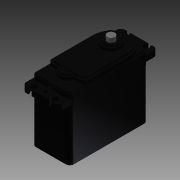
# Autodesk Inventor part: Quarter_scale_servo
Saved by Autodesk Inventor 2015 (Build 190159000, 159)
## iProperties
Created: 2013-11-11
Part Number: Quarter_scale_servo
Material: ABS Plastic
Document SubType Name: Modeling
Designer: 14hensgenw
Density: 1.06 g/cm^3
Appearance: Fine Textured - Black
Author: 14hensgenw
Autodesk Inventor part; units mm, degrees
ref_plane "YZ Plane" through (0, 0, 0) normal (1, 0, 0) x (0, 1, 0)
ref_plane "XZ Plane" through (0, 0, 0) normal (0, 1, 0) x (-1, 0, 0)
sketch "Sketch1" plane through (0, 0, 0) normal (1, 0, 0) x (0, 1, 0)
  line L0 (18.5394, 20.6785) -> (-27.9934, 20.6785)
  line L1 (-27.9934, 20.6785) -> (-27.9934, -37.9701)
  line L2 (-27.9934, -37.9701) -> (18.5394, -37.9701)
  line L3 (18.5394, -37.9701) -> (18.5394, 20.6785)
  point P0 (0, 0)
  dimension "d0" = 58.6486
  dimension "d1" = 46.5328
  constraints: 8 end point, 2 parallel, 1 horizontal, 1 perpendicular
  measures "d0" distance of L2.end L0.start
  measures "d1" distance of L0.start L0.end
extrude "Extrusion1" add sketch "Sketch1" along normal blind 28.4734
sketch "Sketch2" plane through (0, 18.5394, 20.6785) normal (0, 1, 0) x (1, 0, 0)
  line L0 (0, 58.6486) -> (0, 0) projected
  line L1 (0, 0) -> (28.4734, 0) projected
  line L2 (28.4734, 58.6486) -> (28.4734, 0) projected
  line L3 (0, 58.6486) -> (28.4734, 58.6486) projected
  line L4 (1.0287, 58.0708) -> (27.4447, 58.0708)
  line L5 (27.4447, 58.0708) -> (27.4447, 0.5778)
  line L6 (27.4447, 0.5778) -> (1.0287, 0.5778)
  line L7 (1.0287, 0.5778) -> (1.0287, 58.0708)
  line L8 (1.0287, 58.0708) -> (0, 58.0708)
  line L9 (27.4447, 58.0708) -> (28.4734, 58.0708)
  line L10 (14.2367, 58.6486) -> (14.2367, 58.0708)
  line L11 (15.3559, 0) -> (15.3559, 0.5778)
  point P0 (0, 20.6785)
  dimension "d4" = 26.416
  dimension "d5" = 57.4929
  constraints: 16 end point, 4 perpendicular, 4 point on line, 2 equal length, 2 midpoint, 2 parallel, 1 horizontal
  measures "d4" distance of L4.start L4.end
  measures "d5" distance between parallel lines of L6 L4
extrude "Extrusion2" cut sketch "Sketch2" against normal blind 1.016 contours L3 L10 L4 L8 L0 | L8 L7 L6 L11 L1 L0 | L3 L2 L9 L4 L10 | L11 L6 L5 L9 L2 L1
sketch "Sketch3" plane through (1.0287, 18.5394, 20.1007) normal (0, 1, 0) x (1, 0, 0)
  line L0 (0, 0) -> (26.416, 0) projected
  line L1 (0, 57.4929) -> (0, 0) projected
  line L2 (26.416, 57.4929) -> (0, 57.4929) projected
  line L3 (26.416, 0) -> (26.416, 57.4929) projected
  line L4 (27.4447, -0.5778) -> (-1.0287, -0.5778) projected
  line L5 (27.4447, 58.0708) -> (27.4447, -0.5778) projected
  line L6 (-1.0287, 58.0708) -> (27.4447, 58.0708) projected
  line L7 (-1.0287, -0.5778) -> (-1.0287, 58.0708) projected
  circle A0 centre (13.208, 44.4941) radius 13.5767
  line L8 (-0.3683, 44.5981) -> (-1.0287, 44.5981)
  line L9 (26.7843, 44.5981) -> (27.4447, 44.5981)
  line L10 (0, -0.5778) -> (0, 10.8268)
  line L11 (0, 10.8268) -> (-1.0287, 10.8268)
  line L12 (27.4447, 10.8268) -> (-1.0287, 10.8268)
  line L13 (-0.3683, 44.5981) -> (-0.3683, 10.8268)
  line L14 (26.7843, 44.5981) -> (26.7843, 10.8268)
  circle A1 centre (13.208, 12.2237) radius 6.1976
  line L15 (13.208, 10.8268) -> (13.208, 6.0262)
  line L16 (13.208, 6.0262) -> (13.208, 12.2237)
  point P0 (-1.0287, 20.1007)
  dimension "d12" = 12.3952
  dimension "d9" = 0.6604
  dimension "d10" = 11.4046
  dimension "d13" = 4.8006
  constraints: 18 end point, 8 point on line, 6 perpendicular, 2 collinear, 2 point on circle, 1 centre point, 1 midpoint, 1 parallel, 1 tangent, 1 vertical alignment, 2 other
  measures "d9" distance of L8.start L8.end
  measures "d10" distance of L10.start L10.end
  measures "d13" distance of L15.start L15.end
extrude "Extrusion3" add sketch "Sketch3" along normal blind 2.1209 contours L11 L13 A0 L1 | L1 A0 L3 L12 A1 | L3 A0 L14 L12 | A0 L1 | L1 A0 L2 L3 | A1 L12 | L12 L15 A1 | L3 A0 | A1 L15 L12 | A0 L2
sketch "Sketch4" plane through (1.0287, 20.6603, 20.1007) normal (0, 1, 0) x (1, 0, 0)
  line L0 (19.2461, 10.8268) -> (26.7843, 10.8268) projected
  line L1 (26.7843, 10.8268) -> (26.7843, 44.5981) projected
  arc A0 (26.7843, 44.5981) -> (-0.3683, 44.5981) centre (13.208, 44.4941) ccw projected
  line L2 (-0.3683, 44.5981) -> (-0.3683, 10.8268) projected
  line L3 (-0.3683, 10.8268) -> (7.1699, 10.8268) projected
  arc A1 (7.1699, 10.8268) -> (19.2461, 10.8268) centre (13.208, 12.2237) ccw projected
  arc A2 (25.4571, 44.5929) -> (0.9588, 44.5929) centre (13.208, 44.4941) ccw
  line L4 (25.4571, 44.5929) -> (25.4571, 12.1539)
  line L5 (25.4571, 12.1539) -> (18.0779, 12.1539)
  arc A3 (8.3381, 12.1539) -> (18.0779, 12.1539) centre (13.208, 12.2237) ccw
  line L6 (8.3381, 12.1539) -> (0.9588, 12.1539)
  line L7 (0.9588, 12.1539) -> (0.9588, 44.5929)
  point P0 (-1.0287, 20.1007)
  dimension "d18" = 24.4983
  constraints: 8 end point, 4 point on circle, 2 centre point, 5 other
  measures "d18" distance between parallel lines of L4 L7
extrude "Extrusion4" add sketch "Sketch4" along normal blind 1.1176 contours L4 L5 A3 L6 L7 A2
sketch "Sketch5" plane through (1.0287, 21.7779, 20.1007) normal (0, 1, 0) x (1, 0, 0)
  arc A0 (8.3381, 12.1539) -> (18.0779, 12.1539) centre (13.208, 12.2237) ccw projected
  line L0 (25.4571, 12.1539) -> (25.4571, 44.5929) projected
  line L1 (8.3381, 12.1539) -> (18.0779, 12.1539)
  arc A1 (8.3381, 12.1539) -> (18.0779, 12.1539) centre (13.208, 12.2237) ccw
  point P0 (-1.0287, 20.1007)
  constraints: 2 end point, 2 point on circle, 1 centre point, 1 concentric, 1 perpendicular
extrude "Extrusion5" cut sketch "Sketch5" against normal blind 0.4445
fillet "Fillet1" radius 3.175 12 edges at (27.4447, 18.0314, 20.1007) (27.813, 19.5998, 9.2739) (26.4859, 21.2191, 7.9468) (1.9876, 21.2191, 7.9468) (0.6604, 19.5998, 9.2739) (1.0287, 18.0314, 20.1007) (1.0287, 18.0314, -37.3922) (27.4447, 18.0314, -37.3922) (28.4734, -5.235, -37.9701) (28.4734, -5.235, 20.6785) (0, -5.235, -37.9701) (0, -5.235, 20.6785)
ref_plane "Work Plane1" through (0, 14.9072, 20.6785) normal (0, 1, 0) x (1, 0, 0)
sketch "Sketch6" plane through (0, 14.9072, 20.6785) normal (0, 1, 0) x (1, 0, 0)
  arc A0 (0, 3.175) -> (3.175, 0) centre (3.175, 3.175) ccw projected
  line L0 (0, 3.175) -> (0, 55.4736) projected
  arc A1 (3.175, 58.6486) -> (0, 55.4736) centre (3.175, 55.4736) ccw projected
  line L1 (3.175, 58.6486) -> (25.2984, 58.6486) projected
  arc A2 (28.4734, 55.4736) -> (25.2984, 58.6486) centre (25.2984, 55.4736) ccw projected
  line L2 (28.4734, 3.175) -> (28.4734, 55.4736) projected
  arc A3 (25.2984, 0) -> (28.4734, 3.175) centre (25.2984, 3.175) ccw projected
  line L3 (3.175, 0) -> (25.2984, 0) projected
  line L4 (0.3746, 66.2432) -> (28.0988, 66.2432)
  line L5 (28.0988, 66.2432) -> (28.0988, -7.5946)
  line L6 (28.0988, -7.5946) -> (0.3747, -7.5946)
  line L7 (0.3747, -7.5946) -> (0.3746, 66.2432)
  line L8 (14.2367, 58.6486) -> (14.2367, 0)
  line L9 (0.3747, 29.3243) -> (28.0987, 29.3243)
  line L10 (14.2367, -7.5946) -> (14.2367, 29.3243)
  point P0 (0, 20.6785)
  point P1 (14.2367, 29.3243)
  dimension "d23" = 27.7241
  dimension "d24" = 73.8378
  constraints: 14 end point, 7 midpoint, 2 parallel, 1 horizontal, 1 perpendicular
  measures "d23" distance between parallel lines of L5 L7
  measures "d24" distance of L4.end L5.end
extrude "Extrusion6" add sketch "Sketch6" against normal blind 4.0005 contours L7 L9 L8 L3 A0 | A0 L3 L10 L6 L7 | L7 A1 L1 L8 L9 | L7 L4 L5 A2 L1 A1 | L8 L9 L5 A3 L3 | L3 A3 L5 L6 L10 | L8 L1 A2 L5 L9
fillet "Fillet2" radius 3.175 4 edges at (28.0988, 12.9069, 28.2731) (0.3747, 12.9069, 28.2731) (0.3746, 12.9069, -45.5647) (28.0988, 12.9069, -45.5647)
sketch "Sketch7" plane through (0, 14.9072, 20.6785) normal (0, 1, 0) x (1, 0, 0)
  line L0 (3.5497, -7.5946) -> (24.9238, -7.5946) projected
  line L1 (28.0988, -4.4196) -> (28.0988, 1.6788) projected
  line L2 (3.175, 0) -> (25.2984, 0) projected
  line L3 (0.3746, 1.6788) -> (0.3747, -4.4196) projected
  line L4 (4.1592, 0) -> (4.1593, -7.5946)
  line L5 (24.3142, -7.5946) -> (24.3142, 0)
  line L6 (0.3747, -2.5273) -> (28.0988, -2.5273)
  circle A0 centre (6.3183, -4.6863) radius 2.159
  circle A1 centre (22.1552, -4.6863) radius 2.159
  point P0 (0, 20.6785)
  dimension "d28" = 3.7846
  dimension "d29" = 3.7846
  dimension "d30" = 5.0673
  dimension "d31" = 4.318
  dimension "d32" = 4.318
  constraints: 6 end point, 6 point on line, 4 tangent, 3 perpendicular, 2 centre point
  measures "d28" distance between parallel lines of L3 L4
  measures "d29" distance between parallel lines of L1 L5
  measures "d30" distance between parallel lines of L0 L6
  measures "d31" diameter of A0
  measures "d32" diameter of A1
extrude "Extrusion7" cut sketch "Sketch7" against normal blind 4.0005 contours A0 | A1
sketch "Sketch8" plane through (0, 14.9072, 20.6785) normal (0, 1, 0) x (1, 0, 0)
  circle A0 centre (6.3183, -4.6863) radius 2.159 projected
  arc A1 (0.3747, -4.4196) -> (3.5497, -7.5946) centre (3.5497, -4.4196) ccw projected
  line L0 (3.5497, -7.5946) -> (24.9238, -7.5946) projected
  line L1 (3.175, 0) -> (25.2984, 0) projected
  line L2 (0.3746, 1.6788) -> (0.3747, -4.4196) projected
  line L3 (0.3747, -4.4196) -> (0.3747, -8.9936)
  line L4 (0.3747, -7.5946) -> (5.0483, -7.5946)
  line L5 (5.0483, -7.5946) -> (5.0483, -6.4323)
  line L6 (5.0483, -7.5946) -> (7.6772, -7.5946)
  line L7 (7.6772, -7.5946) -> (7.6772, -6.364)
  arc A2 (5.0483, -6.4323) -> (7.6772, -6.364) centre (6.3183, -4.6863) ccw
  line L8 (14.2367, -7.5946) -> (14.2367, 0)
  circle A3 centre (22.1552, -4.6863) radius 2.159
  line L9 (24.9238, -7.5946) -> (3.5497, -7.5946)
  line L10 (28.0988, -7.5946) -> (23.4252, -7.5946)
  line L11 (23.4252, -7.5946) -> (23.4251, -6.4323)
  line L12 (23.4252, -7.5946) -> (20.7963, -7.5946)
  line L13 (20.7963, -7.5946) -> (20.7962, -6.364)
  arc A4 (20.7962, -6.364) -> (23.4251, -6.4323) centre (22.1552, -4.6863) ccw
  point P0 (0, 20.6785)
  dimension "d35" = 4.6736
  dimension "d36" = 2.6289
  constraints: 22 end point, 9 symmetric about line, 8 point on circle, 5 point on line, 3 centre point, 2 midpoint, 2 perpendicular, 1 collinear, 1 concentric, 1 tangent, 2 other
  measures "d35" distance of L4.start L4.end
  measures "d36" distance of L4.end L6.end
extrude "Extrusion8" cut sketch "Sketch8" against normal blind 4.0005 contours A0 L7 L0 L5 | L13 A3 L11 L0
sketch "Sketch9" plane through (0, 14.9072, 20.6785) normal (0, 1, 0) x (1, 0, 0)
  line L0 (7.6772, -7.5946) -> (20.7963, -7.5946) projected
  line L1 (3.175, 0) -> (25.2984, 0) projected
  line L2 (14.2367, 0) -> (14.2367, -7.5946)
  circle A0 centre (14.2367, -3.4163) radius 1.016
  line L3 (13.2207, -3.4163) -> (13.2207, 0)
  line L4 (15.2527, -3.4163) -> (15.2527, 0)
  line L5 (13.2207, 0) -> (15.2527, 0)
  point P0 (0, 20.6785)
  dimension "d39" = 2.032
  dimension "d40" = 3.4163
  constraints: 8 end point, 3 point on line, 2 midpoint, 2 perpendicular, 2 point on circle, 2 tangent, 1 centre point, 1 collinear
  measures "d39" diameter of A0
  measures "d40" distance from line of L1 A0.centre
extrude "Extrusion9" add sketch "Sketch9" along normal blind 1.6383
sketch "Sketch10" plane through (1.0287, 21.7779, 20.1007) normal (0, 1, 0) x (1, 0, 0)
  arc A0 (25.4571, 44.5929) -> (0.9588, 44.5929) centre (13.208, 44.4941) ccw projected
  circle A1 centre (13.208, 44.4941) radius 6.9278
  point P0 (-1.0287, 20.1007)
  dimension "d43" = 13.8557
  constraints: 1 centre point, 1 coincident
  measures "d43" diameter of A1
extrude "Extrusion10" add sketch "Sketch10" along normal blind 1.9558
sketch "Sketch11" plane through (14.2367, 23.7337, -24.3934) normal (0, 1, 0) x (1, 0, 0)
  circle A0 centre (0, 0) radius 6.9278 projected
  circle A1 centre (0, 0) radius 5.461
  point P0 (-14.2367, -24.3934)
  dimension "d46" = 10.922
  constraints: 1 centre point, 1 coincident
  measures "d46" diameter of A1
extrude "Extrusion11" add sketch "Sketch11" along normal blind 0.635 contours A1
sketch "Sketch12" plane through (14.2367, 24.3687, -24.3934) normal (0, 1, 0) x (1, 0, 0)
  circle A0 centre (0, 0) radius 5.461 projected
  circle A1 centre (0, 0) radius 2.8575
  point P0 (-14.2367, -24.3934)
  dimension "d49" = 5.715
  constraints: 1 centre point, 1 coincident
  measures "d49" diameter of A1
extrude "Extrusion12" add sketch "Sketch12" along normal blind 3.2258 contours A1
sketch "Sketch13" plane through (25.2984, -27.9934, -37.9701) normal (0, 0, -1) x (-1, 0, 0)
  line L0 (22.1234, 0) -> (0, 0) projected
  line L1 (22.1234, 38.9001) -> (22.1234, 0) projected
  line L2 (11.0617, 0) -> (11.0617, 3.5687)
  line L3 (11.0617, 3.5687) -> (7.3406, 3.5687)
  line L4 (7.3406, 3.5687) -> (14.7828, 3.5687)
  line L5 (14.7828, 3.5687) -> (14.7828, 7.0485)
  line L6 (14.7828, 7.0485) -> (7.3406, 7.0485)
  line L7 (7.3406, 7.0485) -> (7.3406, 3.5687)
  point P0 (25.2984, 27.9934)
  dimension "d52" = 3.5687
  dimension "d53" = 3.7211
  dimension "d54" = 7.4422
  dimension "d55" = 3.4798
  constraints: 12 end point, 4 parallel, 1 collinear, 1 midpoint, 1 perpendicular
  measures "d52" distance of L2.start L2.end
  measures "d53" distance of L2.end L3.end
  measures "d54" distance of L3.end L4.end
  measures "d55" distance of L4.end L5.end
extrude "Extrusion13" add sketch "Sketch13" along normal blind 6.1214 draft -10
sketch "Sketch14" plane through (1.0287, 18.5394, 20.1007) normal (0, -1, 0) x (1, 0, 0)
  arc A0 (26.7843, -14.0017) -> (26.416, -12.5175) centre (23.6093, -14.0017) ccw projected
  line L0 (26.416, -12.5175) -> (26.416, -47.6366) projected
  arc A1 (26.416, -47.6366) -> (26.7843, -44.5981) centre (13.208, -44.4941) ccw projected
  line L1 (26.7843, -14.0017) -> (26.7843, -44.5981) projected
  point P0 (-1.0287, -20.1007)
extrude "Extrusion14" add sketch "Sketch14" along normal up to next
sketch "Sketch15" plane through (1.0287, 18.5394, 20.1007) normal (0, -1, 0) x (1, 0, 0)
  arc A0 (0, -12.5175) -> (-0.3683, -14.0017) centre (2.8067, -14.0017) ccw projected
  line L0 (-0.3683, -44.5981) -> (-0.3683, -14.0017) projected
  arc A1 (-0.3683, -44.5981) -> (0, -47.6366) centre (13.208, -44.4941) ccw projected
  line L1 (0, -47.6366) -> (0, -12.5175) projected
  point P0 (-1.0287, -20.1007)
extrude "Extrusion15" add sketch "Sketch15" along normal up to next
sketch "Sketch16" plane through (0, 14.9072, 20.6785) normal (0, 1, 0) x (1, 0, 0)
  line L0 (13.2207, 58.6486) -> (13.2207, 62.0649)
  arc A0 (15.2527, 62.0649) -> (13.2207, 62.0649) centre (14.2367, 62.0649) ccw
  line L1 (15.2527, 62.0649) -> (15.2527, 58.6486)
  line L2 (25.2984, 58.6486) -> (15.2527, 58.6486)
  arc A1 (28.0987, 56.9698) -> (25.2984, 58.6486) centre (25.2984, 55.4736) ccw
  line L3 (28.0987, 56.9698) -> (28.0987, 63.0682)
  arc A2 (28.0987, 63.0682) -> (24.9237, 66.2432) centre (24.9237, 63.0682) ccw
  line L4 (24.9237, 66.2432) -> (23.4251, 66.2432)
  line L5 (23.4251, 66.2432) -> (23.4251, 65.0809)
  arc A3 (20.7962, 65.0126) -> (23.4251, 65.0809) centre (22.1551, 63.3349) ccw
  line L6 (20.7962, 65.0126) -> (20.7962, 66.2432)
  line L7 (20.7962, 66.2432) -> (7.6771, 66.2432)
  line L8 (7.6771, 66.2432) -> (7.6771, 65.0126)
  arc A4 (5.0482, 65.0809) -> (7.6771, 65.0126) centre (6.3182, 63.3349) ccw
  line L9 (5.0482, 65.0809) -> (5.0482, 66.2432)
  line L10 (5.0482, 66.2432) -> (3.5496, 66.2432)
  arc A5 (3.5496, 66.2432) -> (0.3746, 63.0682) centre (3.5496, 63.0682) ccw
  line L11 (0.3746, 63.0682) -> (0.3746, 56.9698)
  arc A6 (3.175, 58.6486) -> (0.3746, 56.9698) centre (3.175, 55.4736) ccw
  line L12 (13.2207, 58.6486) -> (3.175, 58.6486)
  arc A7 (28.0988, 63.0682) -> (24.9237, 66.2432) centre (24.9238, 63.0682) ccw projected
  line L13 (24.9237, 66.2432) -> (3.5496, 66.2432) projected
  arc A8 (3.5496, 66.2432) -> (0.3746, 63.0682) centre (3.5496, 63.0682) ccw projected
  line L14 (0.3746, 63.0682) -> (0.3746, 56.9698) projected
  arc A9 (3.175, 58.6486) -> (0.3746, 56.9698) centre (3.175, 55.4736) ccw projected
  line L15 (25.2984, 58.6486) -> (3.175, 58.6486) projected
  arc A10 (28.0988, 56.9698) -> (25.2984, 58.6486) centre (25.2984, 55.4736) ccw projected
  line L16 (28.0988, 56.9698) -> (28.0988, 63.0682) projected
  point P0 (0, 20.6785)
  constraints: 26 end point, 14 point on circle, 7 centre point
extrude "Extrusion16" cut sketch "Sketch16" against normal up to surface (4.0005 mm away) contours L0 A0 L1 L15 | L13 L8 A4 L9 | L5 A3 L6 L13
sketch "Sketch18" plane through (0, 14.9072, 20.6785) normal (0, 1, 0) x (1, 0, 0)
  arc A0 (15.2527, 62.0649) -> (13.2207, 62.0649) centre (14.2367, 62.0649) ccw projected
  line L0 (15.2527, 62.0649) -> (15.2527, 58.6486) projected
  line L1 (13.2207, 58.6486) -> (13.2207, 62.0649) projected
  line L2 (25.2984, 58.6486) -> (15.2527, 58.6486) projected
  line L3 (13.2207, 58.6486) -> (3.175, 58.6486) projected
  line L4 (15.2527, 58.6486) -> (13.2207, 58.6486)
  point P0 (0, 20.6785)
  constraints: 2 end point, 1 horizontal
extrude "Extrusion17" add sketch "Sketch18" along normal blind 1.6383
sketch "Sketch20" plane through (0, 14.9072, 20.6785) normal (0, -1, 0) x (1, 0, 0)
  arc A0 (13.2207, -62.0649) -> (15.2527, -62.0649) centre (14.2367, -62.0649) ccw projected
  line L0 (15.2527, -62.0649) -> (15.2527, -58.6486) projected
  line L1 (13.2207, -58.6486) -> (15.2527, -58.6486) projected
  line L2 (13.2207, -58.6486) -> (13.2207, -62.0649) projected
  point P0 (0, -20.6785)
extrude "Extrusion18" add sketch "Sketch20" along normal up to surface (4.0005 mm away)
body "Solid1"
